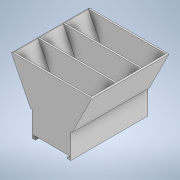
# Autodesk Inventor part: BeadCompartments_3
Saved by Autodesk Inventor 2020 (Build 240168000, 168)
## iProperties
Created: 2021-12-09
Part Number: BeadCompartments_3
Material: Generic
Document SubType Name: Modeling
Designer: danie
Density: 1 g/cm^3
Appearance: Default
Author: danie
Autodesk Inventor part; units mm, degrees
ref_plane "YZ Plane" through (0, 0, 0) normal (1, 0, 0) x (0, 1, 0)
ref_plane "XZ Plane" through (0, 0, 0) normal (0, 1, 0) x (-1, 0, 0)
ref_plane "XY Plane" through (0, 0, 0) normal (0, 0, 1) x (1, 0, 0)
sketch "Sketch1" plane through (0, 0, 0) normal (0, 1, 0) x (-1, 0, 0)
  line L0 (0, 0) -> (-76.2, 0)
  line L1 (-76.2, 0) -> (-76.2, 152.4)
  line L2 (-76.2, 152.4) -> (0, 152.4)
  line L3 (0, 152.4) -> (0, 0)
  line L4 (-3.175, 149.225) -> (-73.025, 149.225)
  line L5 (-73.025, 149.225) -> (-73.025, 3.175)
  line L6 (-73.025, 3.175) -> (-3.175, 3.175)
  line L7 (-3.175, 3.175) -> (-3.175, 149.225)
  dimension "d0" = 76.2
  dimension "d1" = 152.4
  dimension "d2" = 3.175
  constraints: 16 end point, 4 parallel, 2 perpendicular, 1 horizontal, 3 other
  measures "d0" distance of L1.end L2.end
  measures "d1" distance of L0.end L1.end
  measures "d2" distance between parallel lines of L2 L4
extrude "Extrusion1" add sketch "Sketch1" along normal blind 43.815
sketch "Sketch2" plane through (0, 0, 0) normal (0, -1, 0) x (1, 0, 0)
  line L0 (0, 152.4) -> (76.2, 152.4) projected
  line L1 (76.2, 0) -> (0, 0) projected
  line L2 (76.2, 152.4) -> (73.025, 152.4)
  line L3 (73.025, 152.4) -> (73.025, 0)
  line L4 (73.025, 0) -> (76.2, 0)
  line L5 (76.2, 0) -> (76.2, 152.4)
  line L6 (0, 0) -> (3.175, 0)
  line L7 (3.175, 0) -> (3.175, 152.4)
  line L8 (3.175, 152.4) -> (0, 152.4)
  line L9 (0, 152.4) -> (0, 0)
  dimension "d5" = 3.175
  dimension "d6" = 3.175
  constraints: 16 end point, 4 parallel, 2 horizontal, 2 perpendicular, 2 point on line
  measures "d5" distance of L4.end L3.end
  measures "d6" distance of L8.end L7.end
extrude "Extrusion2" add sketch "Sketch2" along normal blind 3.81 contours L0 L7 L1 L9 | L0 L5 L1 L3
sketch "Sketch3" plane through (0, -3.81, 0) normal (0, -1, 0) x (1, 0, 0)
  line L0 (0, 152.4) -> (76.2, 152.4) projected
  line L1 (76.2, 0) -> (0, 0) projected
  line L2 (76.2, 152.4) -> (69.85, 152.4)
  line L3 (69.85, 152.4) -> (69.85, 0)
  line L4 (69.85, 0) -> (76.2, 0)
  line L5 (76.2, 0) -> (76.2, 152.4)
  line L6 (0, 152.4) -> (6.35, 152.4)
  line L7 (6.35, 152.4) -> (6.35, 0)
  line L8 (6.35, 0) -> (0, 0)
  line L9 (0, 0) -> (0, 152.4)
  dimension "d9" = 6.35
  dimension "d10" = 6.35
  constraints: 16 end point, 4 parallel, 2 horizontal, 2 perpendicular, 2 point on line
  measures "d9" distance of L4.end L3.end
  measures "d10" distance of L7.end L8.end
extrude "Extrusion3" add sketch "Sketch3" along normal blind 3.175 contours L0 L7 L1 L9 | L0 L5 L1 L3
sketch "Sketch4" plane through (73.025, 0, 0) normal (0, 0, -1) x (-1, 0, 0)
  line L0 (0, -3.81) -> (3.175, -3.81) projected
  line L1 (73.025, -6.985) -> (66.675, -6.985) projected
  line L2 (3.175, -3.81) -> (66.675, -3.81)
  line L3 (66.675, -3.81) -> (66.675, -6.985)
  line L4 (66.675, -6.985) -> (3.175, -6.985)
  line L5 (3.175, -6.985) -> (3.175, -3.81)
  point P0 (73.025, 0)
  constraints: 8 end point, 2 parallel, 1 horizontal, 1 perpendicular
extrude "Extrusion4" add sketch "Sketch4" against normal blind 3.175
sketch "Sketch5" plane through (3.175, 0, 3.175) normal (1, 0, 0) x (0, 0, -1)
  line L0 (-146.05, 0) -> (-146.05, 43.815) construction
  line L1 (-146.05, 43.815) -> (-99.568, 43.815) construction
  line L2 (-146.05, 43.815) -> (0, 43.815) construction
  line L3 (-99.568, 43.815) -> (-96.393, 43.815) construction
  line L4 (-96.393, 43.815) -> (-49.657, 43.815) construction
  line L5 (-49.657, 43.815) -> (-46.482, 43.815) construction
  line L6 (0, 0) -> (0, 43.815) construction
  line L7 (-46.482, 43.815) -> (0, 43.815) construction
  line L8 (-46.482, 43.815) -> (0, 43.815) construction
  line L9 (-46.482, 43.815) -> (0, 43.815) construction
  line L10 (-99.568, 43.815) -> (-96.393, 43.815)
  line L11 (-96.393, 43.815) -> (-96.393, 0)
  line L12 (-96.393, 0) -> (-99.568, 0)
  line L13 (-99.568, 0) -> (-99.568, 43.815)
  line L14 (-49.657, 43.815) -> (-46.482, 43.815)
  line L15 (-46.482, 43.815) -> (-46.482, 0)
  line L16 (-46.482, 0) -> (-49.657, 0)
  line L17 (-49.657, 0) -> (-49.657, 43.815)
  point P0 (3.175, 0)
  dimension "d15" = 46.482
  dimension "d16" = 3.175
  dimension "d17" = 46.736
  dimension "d18" = 3.175
  dimension "d19" = 43.815
  dimension "d20" = 43.815
  constraints: 30 end point, 4 parallel, 4 point on line, 3 perpendicular, 2 collinear, 2 horizontal
  measures "d15" distance of L0.end L1.end
  measures "d16" distance of L1.end L3.end
  measures "d17" distance of L3.end L4.end
  measures "d18" distance of L4.end L5.end
  measures "d19" distance of L10.end L11.end
  measures "d20" distance of L14.end L15.end
extrude "Extrusion5" add sketch "Sketch5" along normal up to next
sketch "Sketch6" plane through (3.175, 0, 152.4) normal (0, 0, 1) x (1, 0, 0)
  line L0 (73.025, 43.815) -> (-3.175, 43.815) projected
  line L1 (-3.175, 43.815) -> (73.025, 43.815)
  line L2 (73.025, 43.815) -> (73.025, 120.015)
  line L3 (73.025, 120.015) -> (-3.175, 120.015)
  line L4 (-3.175, 120.015) -> (-3.175, 43.815)
  point P0 (-3.175, 0)
  dimension "d23" = 76.2
  constraints: 8 end point, 2 parallel, 1 horizontal, 1 perpendicular
  measures "d23" distance of L2.end L1.end
extrude "Extrusion6" add sketch "Sketch6" against normal blind 3.175
sketch "Sketch7" plane through (3.175, 0, 152.4) normal (0, 0, 1) x (1, 0, 0)
  line L0 (73.025, 120.015) -> (73.025, 43.815) projected
  line L1 (73.025, 120.015) -> (111.125, 120.015)
  line L2 (73.025, 43.815) -> (111.125, 120.015)
  line L3 (73.025, 120.015) -> (-3.175, 120.015) projected
  line L4 (-3.175, 120.015) -> (-41.275, 120.015)
  line L5 (-3.175, 120.015) -> (34.925, 120.015) construction
  line L6 (-3.175, 43.815) -> (-3.175, 120.015) projected
  line L7 (-41.275, 120.015) -> (-3.175, 43.815)
  point P0 (-3.175, 0)
  dimension "d26" = 38.1
  dimension "d27" = 38.1
  dimension "d28" = 180
  constraints: 10 end point, 3 horizontal, 1 collinear
  measures "d26" distance of L0.start L1.end
  measures "d27" distance of L3.end L4.end
  measures "d28" angle of L4 L5
extrude "Extrusion7" add sketch "Sketch7" against normal blind 3.175
sketch "Sketch8" plane through (76.2, 43.815, 0) normal (0, 0, -1) x (-1, 0, 0)
  line L0 (3.175, 0) -> (0, 0) projected
  line L1 (0, 0) -> (-38.1, 76.2)
  line L2 (114.3, 76.2) -> (-38.1, 76.2) projected
  line L3 (-38.1, 76.2) -> (114.3, 76.2)
  line L4 (76.2, 0) -> (73.025, 0) projected
  line L5 (114.3, 76.2) -> (76.2, 0)
  line L6 (0, 0) -> (76.2, 0)
  line L7 (73.025, 0) -> (3.175, 0) projected
  point P0 (76.2, -43.815)
  constraints: 8 end point, 2 collinear
extrude "Extrusion8" add sketch "Sketch8" against normal blind 3.175
sketch "Sketch9" plane through (76.2, 43.815, 152.4) normal (0.8944, -0.4472, 0) x (0, 0, -1)
  line L0 (0, 85.1942) -> (3.175, 85.1942) projected
  line L1 (152.4, 85.1942) -> (152.4, 0) projected
  line L2 (0, 85.1942) -> (152.4, 85.1942)
  line L3 (152.4, 85.1942) -> (152.4, 0)
  line L4 (152.4, 0) -> (0, 0)
  line L5 (0, 0) -> (0, 85.1942)
  point P0 (152.4, -73.267)
  constraints: 8 end point, 2 parallel, 1 horizontal, 1 perpendicular
extrude "Extrusion9" add sketch "Sketch9" along normal blind 3.175
sketch "Sketch10" plane through (0, 43.815, 0) normal (-0.8944, -0.4472, 0) x (0, 0, 1)
  line L0 (0, 85.1942) -> (3.175, 85.1942) projected
  line L1 (152.4, -45.4369) -> (152.4, 0) projected
  line L2 (0, 85.1942) -> (152.4, 85.1942)
  line L3 (152.4, 85.1942) -> (152.4, 0)
  line L4 (152.4, 0) -> (0, 0)
  line L5 (0, 0) -> (0, 85.1942)
  point P0 (0, -39.1893)
  constraints: 8 end point, 2 parallel, 1 horizontal, 1 perpendicular
extrude "Extrusion10" add sketch "Sketch10" along normal blind 3.175
sketch "Sketch11" plane through (114.3, 120.015, 152.4) normal (0, 1, 0) x (1, 0, 0)
  line L0 (-111.125, 49.657) -> (-41.275, 49.657) construction
  line L1 (-111.125, 49.657) -> (-152.4, 49.657) construction
  line L2 (-152.4, 3.175) -> (-152.4, 149.225) construction
  line L3 (-111.125, 52.832) -> (-41.275, 52.832) construction
  line L4 (-41.275, 52.832) -> (0, 52.832) construction
  line L5 (0, 149.225) -> (0, 3.175) construction
  line L6 (-111.125, 99.568) -> (-41.275, 99.568) construction
  line L7 (-111.125, 99.568) -> (-152.4, 99.568) construction
  line L8 (-111.125, 102.743) -> (-41.275, 102.743) construction
  line L9 (-41.275, 102.743) -> (0, 102.743) construction
  line L10 (-152.4, 49.657) -> (0, 49.657)
  line L11 (0, 49.657) -> (0, 52.832)
  line L12 (0, 52.832) -> (-152.4, 52.832)
  line L13 (-152.4, 52.832) -> (-152.4, 49.657)
  line L14 (-152.4, 99.568) -> (0, 99.568)
  line L15 (0, 99.568) -> (0, 102.743)
  line L16 (0, 102.743) -> (-152.4, 102.743)
  line L17 (-152.4, 102.743) -> (-152.4, 99.568)
  point P0 (-114.3, 152.4)
  constraints: 24 end point, 4 horizontal, 4 parallel, 4 point on line, 3 perpendicular, 1 collinear
extrude "Extrusion11" add sketch "Sketch11" against normal blind 3.175
sketch "Sketch12" plane through (-38.1, 120.015, 102.743) normal (0, 0, 1) x (1, 0, 0)
  line L0 (150.8125, -3.175) -> (1.5875, -3.175) projected
  line L1 (1.5875, -3.175) -> (38.1, -76.2)
  line L2 (38.1, -76.2) -> (114.3, -76.2)
  line L3 (152.4, 0) -> (150.8125, -3.175) projected
  line L4 (114.3, -76.2) -> (150.8125, -3.175)
  line L5 (150.8125, -3.175) -> (1.5875, -3.175)
  point P0 (38.1, -120.015)
  constraints: 8 end point, 1 collinear, 1 horizontal, 1 parallel
extrude "Extrusion12" add sketch "Sketch12" against normal blind 3.175
sketch "Sketch13" plane through (-38.1, 120.015, 52.832) normal (0, 0, 1) x (1, 0, 0)
  line L0 (150.8125, -3.175) -> (1.5875, -3.175) projected
  line L1 (1.5875, -3.175) -> (38.1, -76.2)
  line L2 (38.1, -76.2) -> (114.3, -76.2)
  line L3 (152.4, 0) -> (150.8125, -3.175) projected
  line L4 (114.3, -76.2) -> (150.8125, -3.175)
  line L5 (150.8125, -3.175) -> (1.5875, -3.175)
  point P0 (38.1, -120.015)
  constraints: 8 end point, 1 collinear, 1 horizontal, 1 parallel
extrude "Extrusion13" add sketch "Sketch13" against normal blind 3.175
sketch "Sketch14" plane through (3.175, 0, 152.4) normal (0, 0, 1) x (1, 0, 0)
  line L0 (-3.175, 43.815) -> (-6.0148, 42.3951) projected
  line L1 (-6.0148, 42.3951) -> (-3.175, 42.3951)
  line L2 (-3.175, 43.815) -> (-3.175, -6.985) projected
  line L3 (-3.175, 42.3951) -> (-3.175, 43.815)
  line L4 (-3.175, 43.815) -> (-6.0148, 42.3951)
  line L5 (75.8648, 42.3951) -> (73.025, 42.3951)
  line L6 (73.025, -6.985) -> (73.025, 43.815) projected
  line L7 (73.025, 42.3951) -> (73.025, 43.815)
  line L8 (73.025, 43.815) -> (75.8648, 42.3951)
  line L9 (73.025, 43.815) -> (75.8648, 42.3951) projected
  point P0 (-3.175, 0)
  constraints: 12 end point, 2 perpendicular, 2 point on line, 1 collinear, 1 horizontal
extrude "Extrusion14" add sketch "Sketch14" against normal blind 152.4
body "Solid1"
